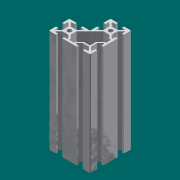
# Autodesk Inventor part: HFS5-404020-100
Saved by Autodesk Inventor 2016 (Build 200138000, 138)
## iProperties
Category: PARTsolutions
Company: MISUMI
Created: 2016-02-10
Part Number: HFS5-404020-100
Catalog Web Link: www.cadenas.de
Description: HFS30A5-20, HFS45A5-20, HFS60A5-20, HFS5-404020, HFSR5-404020, HFSR5-2020-HFS5 Series Aluminum Extrusions 20mm Square -Other Shapes-
Vendor: MISUMI
Document SubType Name: Modeling
Designer: psAdmin
Manufacturer: MISUMI
Mass: 114.059 g
Surface Area: 436.475 cm^2
Volume: 42.244 cm^3
Density: 2.7 g/cm^3
Material: Aluminum 6061
Appearance: Aluminum - Flat
PSOL_IDENT_0: {$CADENAS_DATA\23d-libs\misumi\metric\38_al_extrusions_blackets\5\hfs30a5_20.prj},449 {VTYP=3D},{NB=
PSOL_IDENT_1: HFS5-404020-100},{LINA=HFS5-404020-100},{NN=HFS30A5-20, HFS45A5-20, HFS60A5-20, HFS5-404020, HFSR5-4
PSOL_IDENT_2: 04020, HFSR5-2020},{DATE=17.07.2015 10:47:06},{GEOMDATE=28.01.2015 05:29:00},{VERSION=},{LINEID=140}
PSOL_IDENT_3: ,{LINESUBID=-1},{WBVAR=L,ALT1,ALT2,ALT4,ALT5,CP5,DL5,DR5,ALT6,ALT9,ALT10,ALT11,HP6,NHL6,DL6,NHR6,DR6
PSOL_IDENT_4: ,ALT7,ALT8,NH9,AH,BH,CH,DH,EH,NH10,AV,BV,CV,DV,EV,NH11,AP,BP,CP,DP,EP,ALT16,HP16,DL16,DR16,ALT17,HQ1
PSOL_IDENT_5: 7,JLP,ALT18,HQ18,KLP,ALT19,ALT20}  {NB=HFS5-404020-100},{LINA=HFS5-404020-100},{KT=DUMMY},{PN=HFS5-4
PSOL_IDENT_6: 04020-100},{TPS=HFS5-404020},{MAT=A6N01SS-T5 Aluminum Alloy},{ST=Clear Anodize},{FRMW=40},{FRMH=40},
PSOL_IDENT_7: {FRD=4.2},{L=100},{MASS=1.16},{SA=429},{LX=6.61x10^4},{LY=6.61x10^4},{ALT1=},{M1=0},{DPL1=0},{DPR1=0
PSOL_IDENT_8: },{ALT1PN=},{ALT2=},{ALT2ALG= '','w/o End Tapping (Heli-Coil Insert)','LHP','with LHP (Tapping on th
PSOL_IDENT_9: e Left (Heli-Coil Insert))','RHP','with RHP (Tapping on the Right (Heli-Coil Insert))','HPW','with H
PSOL_IDENT_10: PW (Tapping on Both Ends (Heli-Coil Insert))' },{M2=0},{DP2=0},{ALT2PN=},{ALT4=},{ALT4ALG= '', 'w/o
PSOL_IDENT_11: SC (High Precision Cut)', 'SC', 'with SC (High Precision Cut)' },{ALT4PN=},{ALT5=},{ALT5ALG= '','w/o
PSOL_IDENT_12: 45 Degree Cut','1','with 45 Degree Cut' },{CP5=},{CP5ALG= '','N/A' },{DL5=},{DL5ALG= '','N/A' },{DR
PSOL_IDENT_13: 5=},{DR5ALG= '','N/A' },{FRMLALT5=0},{FRMRALT5=0},{RA5=0},{ALT5PN=},{ALT6=},{ALT6ALG= '','w/o Fasten
PSOL_IDENT_14: ing Location Wrench Access Hole Alterations','1','with Fastening Location Wrench Access Hole Alterat
PSOL_IDENT_15: ions' },{ALT9=},{ALT9ALG= '','w/o Location Specified Wrench Access Hole Alteratons (Horizontal)','1'
PSOL_IDENT_16: ,'with Location Specified Wrench Access Hole Alteratons (Horizontal)' },{ALT10=},{ALT10ALG= '','w/o
PSOL_IDENT_17: Location Specified Wrench Access Hole Alteratons (Vertical)','1','with Location Specified Wrench Acc
PSOL_IDENT_18: ess Hole Alteratons (Vertical)' },{ALT11=},{ALT11ALG= '','w/o Location Specified Wrench Access Hole
PSOL_IDENT_19: Alteratons (Crisscross)','1','with Location Specified Wrench Access Hole Alteratons (Crisscross)' },
PSOL_IDENT_20: {HP6=},{HP6ALG= '','N/A' },{NHL6=},{NHL6ALG= '','N/A' },{DL6=},{DL6ALG= '','N/A' },{NHR6=},{NHR6ALG=
PSOL_IDENT_21: '','N/A' },{DR6=},{DR6ALG= '','N/A' },{HL6=0},{HL6D=0},{HR6=0},{HR6D=0},{J6=0},{J6D=0},{K6=0},{K6D=
PSOL_IDENT_22: 0},{DD6=0.00},{DD6ALG=0},{ALT7=},{ALT7ALG= '','N/A' },{ALT8=},{ALT8ALG= '','N/A' },{ALT678PN=},{NH9=
PSOL_IDENT_23: 0},{NH9MAX=5},{NH9ALG=[0]},{AH=0.0},{AHMIN=7},{AHMAX=95},{AHALG=[0]},{BH=0.0},{BHMIN=2},{BHMAX=97},{
PSOL_IDENT_24: BHALG=[0]},{CH=0.0},{CHMIN=2},{CHMAX=99},{CHALG=[0]},{DH=0.0},{DHMIN=2},{DHMAX=101},{DHALG=[0]},{EH=
PSOL_IDENT_25: 0.0},{EHMIN=2},{EHMAX=93},{EHALG=[0]},{NH10=0},{NH10MAX=5},{NH10ALG=[0]},{AV=0.0},{AVMIN=7},{AVMAX=9
PSOL_IDENT_26: 5},{AVALG=[0]},{BV=0.0},{BVMIN=2},{BVMAX=97},{BVALG=[0]},{CV=0.0},{CVMIN=2},{CVMAX=99},{CVALG=[0]},{
PSOL_IDENT_27: DV=0.0},{DVMIN=2},{DVMAX=101},{DVALG=[0]},{EV=0.0},{EVMIN=2},{EVMAX=93},{EVALG=[0]},{NH11=0},{NH11MA
PSOL_IDENT_28: X=5},{NH11ALG=[0]},{AP=0.0},{APMIN=7},{APMAX=95},{APALG=[0]},{BP=0.0},{BPMIN=2},{BPMAX=97},{BPALG=[0
PSOL_IDENT_29: ]},{CP=0.0},{CPMIN=2},{CPMAX=99},{CPALG=[0]},{DP=0.0},{DPMIN=2},{DPMAX=101},{DPALG=[0]},{EP=0.0},{EP
PSOL_IDENT_30: MIN=2},{EPMAX=93},{EPALG=[0]},{ALT9PN=},{ALT10PN=},{ALT11PN=},{ALT91011PN=},{ALT16=},{ALT16ALG= '','
PSOL_IDENT_31: w/o M Type Hole Alteration','1','with M Type Hole Alteration' },{HP16=},{HP16ALG= '','N/A' },{DL16=}
PSOL_IDENT_32: ,{DL16ALG= '','N/A' },{DR16=},{DR16ALG= '','N/A' },{H116=0},{D16=0.0},{ALT16PN=},{ALT17=},{ALT17ALG=
PSOL_IDENT_33: '','w/o L Type Hole Alteration (Top)','1','with L Type Hole Alteration (Top)' },{HQ17=0},{HQ17ALG=0
PSOL_IDENT_34: },{JLP=0},{JLPMIN=4.9},{JLPMAX=0},{JLPALG=[0]},{L17=0},{D17=0.0},{ALT18=},{ALT18ALG= '','w/o L Type
PSOL_IDENT_35: Hole Alteration (Bottom)','1','with L Type Hole Alteration (Bottom)' },{HQ18=0},{HQ18ALG=0},{KLP=0},
PSOL_IDENT_36: {KLPMIN=4.9},{KLPMAX=0},{KLPALG=[0]},{L18=0},{D18=0.0},{ALT1718PN=},{ALT19=},{ALT19ALG= '','N/A' },{
PSOL_IDENT_37: M19=0},{DP19=0},{ALT19PN=},{ALT20=},{ALT20PN=},{ERRORALT01=OK},{ERRORALT02=OK},{ERRORALT05=OK},{ERRO
PSOL_IDENT_38: RALT06091=OK},{ERRORALT06092=OK},{ERRORALT06093=OK},{ERRORALT06094=OK},{ERRORALT06101=OK},{ERRORALT0
PSOL_IDENT_39: 6102=OK},{ERRORALT06103=OK},{ERRORALT06104=OK},{ERRORALT06111=OK},{ERRORALT06112=OK},{ERRORALT06113=
PSOL_IDENT_40: OK},{ERRORALT06114=OK},{ERRORALT0616=OK},{ERRORALT06171=OK},{ERRORALT06172=OK},{ERRORALT06173=OK},{E
PSOL_IDENT_41: RRORALT06181=OK},{ERRORALT06182=OK},{ERRORALT06183=OK},{ERRORALT0619=OK},{ERRORALT0911=OK},{ERRORALT
PSOL_IDENT_42: 0916=OK},{ERRORALT0917=OK},{ERRORALT0918=OK},{ERRORALT0919=OK},{ERRORALT1011=OK},{ERRORALT1016=OK},{
PSOL_IDENT_43: ERRORALT1017=OK},{ERRORALT1018=OK},{ERRORALT1019=OK},{ERRORALT1116=OK},{ERRORALT1117=OK},{ERRORALT11
PSOL_IDENT_44: 18=OK},{ERRORALT1119=OK},{ERRORALT1617=OK},{ERRORALT1618=OK},{ERRORALT1619=OK},{ERRORALT1719=OK},{ER
PSOL_IDENT_45: RORALT1819=OK},{ERRORPN=},{TFW=0},{IDM1=3.242}
NN: HFS30A5-20, HFS45A5-20, HFS60A5-20, HFS5-404020, HFSR5-404020, HFSR5-2020
NT: HFS5 Series Aluminum Extrusions 20mm Square -Other Shapes-
NB: HFS5-404020-100
NBSYN: $PN.
LINA: HFS5-404020-100
PN: HFS5-404020-100
TPS: HFS5-404020
MAT: A6N01SS-T5 Aluminum Alloy
ST: Clear Anodize
L: 100
MASS: 1.16
SA: 429
LX: 6.61x10^4
LY: 6.61x10^4
ALT1: w/o End Tapping
M1: 0
DPL1: 0
DPR1: 0
ALT2: w/o End Tapping (Heli-Coil Insert)
M2: 0
DP2: 0
ALT4: w/o SC (High Precision Cut)
ALT5: w/o 45 Degree Cut
CP5: N/A
DL5: N/A
DR5: N/A
ALT6: w/o Fastening Location Wrench Access Hole Alterations
ALT9: w/o Location Specified Wrench Access Hole Alteratons (Horizontal)
ALT10: w/o Location Specified Wrench Access Hole Alteratons (Vertical)
ALT11: w/o Location Specified Wrench Access Hole Alteratons (Crisscross)
HP6: N/A
NHL6: N/A
DL6: N/A
NHR6: N/A
DR6: N/A
HL6D: 0
HR6D: 0
J6D: 0
K6D: 0
DD6: 0.00
ALT7: N/A
ALT8: N/A
NH9: 0
AH: 0.0
BH: 0.0
CH: 0.0
DH: 0.0
EH: 0.0
NH10: 0
AV: 0.0
BV: 0.0
CV: 0.0
DV: 0.0
EV: 0.0
NH11: 0
AP: 0.0
BP: 0.0
CP: 0.0
DP: 0.0
EP: 0.0
ALT16: w/o M Type Hole Alteration
HP16: N/A
DL16: N/A
DR16: N/A
H116: 0
D16: 0.0
ALT17: w/o L Type Hole Alteration (Top)
HQ17: 0
JLP: 0
D17: 0.0
ALT18: w/o L Type Hole Alteration (Bottom)
HQ18: 0
KLP: 0
D18: 0.0
ALT19: N/A
M19: 0
ALT20: w/o CW (End Face C Chamfering)
SUPPLIER: MISUMI
ARTICLENO: HFS5-404020-100
BOMINFO: HFS5-404020-100
CREATOR: CADENAS GmbH
Title: HFS5-404020-100
Author: Cadenas PARTsolutions
Comments: HFS5 Series Aluminum Extrusions 20mm Square -Other Shapes-
Autodesk Inventor part; units mm, degrees
ref_plane "YZ Plane" through (0, 0, 0) normal (1, 0, 0) x (0, 1, 0)
ref_plane "XZ Plane" through (0, 0, 0) normal (0, 1, 0) x (-1, 0, 0)
ref_plane "XY Plane" through (0, 0, 0) normal (0, 0, 1) x (1, 0, 0)
sketch "Sketch_1" plane through (0, 0, 0) normal (0, 0, 1) x (1, 0, 0)
  line L0 (-40, 7) -> (-40, 1)
  arc A0 (-40, 1) -> (-39, 0) centre (-39, 1) ccw
  line L1 (-39, 0) -> (-33, 0)
  line L2 (-33, 0) -> (-33, 2)
  line L3 (-33, 2) -> (-36, 2)
  line L4 (-36, 2) -> (-36, 2.9393)
  line L5 (-36, 2.9393) -> (-32.9393, 6)
  line L6 (-32.9393, 6) -> (-30.5196, 6)
  line L7 (-30.5196, 6) -> (-30, 6.3)
  line L8 (-30, 6.3) -> (-29.4804, 6)
  line L9 (-29.4804, 6) -> (-27.0607, 6)
  line L10 (-27.0607, 6) -> (-24, 2.9393)
  line L11 (-24, 2.9393) -> (-24, 2)
  line L12 (-24, 2) -> (-27, 2)
  line L13 (-27, 2) -> (-27, 0)
  line L14 (-27, 0) -> (-13, 0)
  line L15 (-13, 0) -> (-13, 2)
  line L16 (-13, 2) -> (-16, 2)
  line L17 (-16, 2) -> (-16, 2.9393)
  line L18 (-16, 2.9393) -> (-12.9393, 6)
  line L19 (-12.9393, 6) -> (-7.0607, 6)
  line L20 (-7.0607, 6) -> (-4, 2.9393)
  line L21 (-4, 2.9393) -> (-4, 2)
  line L22 (-4, 2) -> (-7, 2)
  line L23 (-7, 2) -> (-7, 0)
  line L24 (-7, 0) -> (-1, 0)
  arc A1 (-1, 0) -> (0, 1) centre (-1, 1) ccw
  line L25 (0, 1) -> (0, 7)
  line L26 (0, 7) -> (-2, 7)
  line L27 (-2, 7) -> (-2, 4)
  line L28 (-2, 4) -> (-2.9393, 4)
  line L29 (-2.9393, 4) -> (-6, 7.0607)
  line L30 (-6, 7.0607) -> (-6, 12.9393)
  line L31 (-6, 12.9393) -> (-2.9393, 16)
  line L32 (-2.9393, 16) -> (-2, 16)
  line L33 (-2, 16) -> (-2, 13)
  line L34 (-2, 13) -> (0, 13)
  line L35 (0, 13) -> (0, 27)
  line L36 (0, 27) -> (-2, 27)
  line L37 (-2, 27) -> (-2, 24)
  line L38 (-2, 24) -> (-2.9393, 24)
  line L39 (-2.9393, 24) -> (-6, 27.0607)
  line L40 (-6, 27.0607) -> (-6, 29.4804)
  line L41 (-6, 29.4804) -> (-6.3, 30)
  line L42 (-6.3, 30) -> (-6, 30.5196)
  line L43 (-6, 30.5196) -> (-6, 32.9393)
  line L44 (-6, 32.9393) -> (-2.9393, 36)
  line L45 (-2.9393, 36) -> (-2, 36)
  line L46 (-2, 36) -> (-2, 33)
  line L47 (-2, 33) -> (0, 33)
  line L48 (0, 33) -> (0, 39)
  arc A2 (0, 39) -> (-1, 40) centre (-1, 39) ccw
  line L49 (-1, 40) -> (-7, 40)
  line L50 (-7, 40) -> (-7, 38)
  line L51 (-7, 38) -> (-4, 38)
  line L52 (-4, 38) -> (-4, 37.0607)
  line L53 (-4, 37.0607) -> (-7.0607, 34)
  line L54 (-7.0607, 34) -> (-9.4804, 34)
  line L55 (-9.4804, 34) -> (-10, 33.7)
  line L56 (-10, 33.7) -> (-10.5196, 34)
  line L57 (-10.5196, 34) -> (-12.9393, 34)
  line L58 (-12.9393, 34) -> (-16, 37.0607)
  line L59 (-16, 37.0607) -> (-16, 38)
  line L60 (-16, 38) -> (-13, 38)
  line L61 (-13, 38) -> (-13, 40)
  line L62 (-13, 40) -> (-19, 40)
  arc A3 (-19, 40) -> (-20, 39) centre (-19, 39) ccw
  line L63 (-20, 39) -> (-20, 33)
  line L64 (-20, 33) -> (-18, 33)
  line L65 (-18, 33) -> (-18, 36)
  line L66 (-18, 36) -> (-17.0607, 36)
  line L67 (-17.0607, 36) -> (-14, 32.9393)
  line L68 (-14, 32.9393) -> (-14, 30.5196)
  line L69 (-14, 30.5196) -> (-13.7, 30)
  line L70 (-13.7, 30) -> (-14, 29.4804)
  line L71 (-14, 29.4804) -> (-14, 27.0607)
  line L72 (-14, 27.0607) -> (-17.0607, 24)
  line L73 (-17.0607, 24) -> (-18, 24)
  line L74 (-18, 24) -> (-18, 27)
  line L75 (-18, 27) -> (-20, 27)
  line L76 (-20, 27) -> (-20, 20.3)
  arc A4 (-20.3, 20) -> (-20, 20.3) centre (-20.3, 20.3) ccw
  line L77 (-20.3, 20) -> (-27, 20)
  line L78 (-27, 20) -> (-27, 18)
  line L79 (-27, 18) -> (-24, 18)
  line L80 (-24, 18) -> (-24, 17.0607)
  line L81 (-24, 17.0607) -> (-27.0607, 14)
  line L82 (-27.0607, 14) -> (-29.4804, 14)
  line L83 (-29.4804, 14) -> (-30, 13.7)
  line L84 (-30, 13.7) -> (-30.5196, 14)
  line L85 (-30.5196, 14) -> (-32.9393, 14)
  line L86 (-32.9393, 14) -> (-36, 17.0607)
  line L87 (-36, 17.0607) -> (-36, 18)
  line L88 (-36, 18) -> (-33, 18)
  line L89 (-33, 18) -> (-33, 20)
  line L90 (-33, 20) -> (-39, 20)
  arc A5 (-39, 20) -> (-40, 19) centre (-39, 19) ccw
  line L91 (-40, 19) -> (-40, 13)
  line L92 (-40, 13) -> (-38, 13)
  line L93 (-38, 13) -> (-38, 16)
  line L94 (-38, 16) -> (-37.0607, 16)
  line L95 (-37.0607, 16) -> (-34, 12.9393)
  line L96 (-34, 12.9393) -> (-34, 10.5196)
  line L97 (-34, 10.5196) -> (-33.7, 10)
  line L98 (-33.7, 10) -> (-34, 9.4804)
  line L99 (-34, 9.4804) -> (-34, 7.0607)
  line L100 (-34, 7.0607) -> (-37.0607, 4)
  line L101 (-37.0607, 4) -> (-38, 4)
  line L102 (-38, 4) -> (-38, 7)
  line L103 (-38, 7) -> (-40, 7)
  line L104 (-26, 12.9393) -> (-26, 7.0607)
  line L105 (-26, 7.0607) -> (-22.5, 3.5607)
  line L106 (-22.5, 3.5607) -> (-22.5, 2)
  line L107 (-22.5, 2) -> (-17.5, 2)
  line L108 (-17.5, 2) -> (-17.5, 3.5607)
  line L109 (-17.5, 3.5607) -> (-13.5607, 7.5)
  line L110 (-13.5607, 7.5) -> (-7.5, 7.5)
  line L111 (-7.5, 7.5) -> (-7.5, 13.5607)
  line L112 (-7.5, 13.5607) -> (-3.5607, 17.5)
  line L113 (-3.5607, 17.5) -> (-2, 17.5)
  line L114 (-2, 17.5) -> (-2, 22.5)
  line L115 (-2, 22.5) -> (-3.5607, 22.5)
  line L116 (-3.5607, 22.5) -> (-7.0607, 26)
  line L117 (-7.0607, 26) -> (-12.9393, 26)
  line L118 (-12.9393, 26) -> (-26, 12.9393)
  constraints: 238 end point, 12 point on circle, 6 centre point
extrude "Extrusion1" add sketch "Sketch_1" against normal blind 100
sketch "Sketch2" plane through (0, 0, -100) normal (0, 0, -1) x (-1, 0, 0)
  point P0 (10, 30)
hole "Hole1" at (-10, 30, -100) direction (0, 0, 1) diameter 4.2 depth 100
sketch "Sketch3" plane through (0, 0, -100) normal (0, 0, -1) x (-1, 0, 0)
  point P0 (30, 10)
hole "Hole2" at (-30, 10, -100) direction (0, 0, 1) diameter 4.2 depth 100
body "Solid1"
